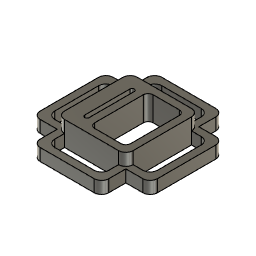
tv-foot-crt (Autodesk Fusion 360 design; units mm, degrees)
Autodesk Fusion 360 part; units mm, degrees
sketch "Sketch1" plane through (0, 0, 0) normal (0, 0, 1) x (1, 0, 0)
  line L0 (0, 0) -> (70.5, 0)
  line L1 (70.5, 0) -> (70.5, 75)
  line L2 (70.5, 75) -> (0, 75)
  line L3 (0, 75) -> (0, 0)
  line L4 (70.5, 0) -> (415.5625, 0) construction
  line L5 (16.25, 75) -> (16.25, 0) construction
  line L6 (14, 60.75) -> (14, 14.25)
  arc A0 (14, 14.25) -> (18.5, 14.25) centre (16.25, 14.25) ccw
  line L7 (18.5, 14.25) -> (18.5, 60.75)
  arc A1 (18.5, 60.75) -> (14, 60.75) centre (16.25, 60.75) ccw
  line L8 (16.25, 63) -> (16.25, 12) construction
  line L9 (12, 60.75) -> (12, 14.25)
  arc A2 (12, 14.25) -> (20.5, 14.25) centre (16.25, 14.25) ccw
  line L10 (20.5, 14.25) -> (20.5, 60.75)
  arc A3 (20.5, 60.75) -> (12, 60.75) centre (16.25, 60.75) ccw
  line L11 (8, 0) -> (8, 75)
  dimension "d3" = 75
  dimension "d10" = 4.5
  dimension "d13" = 2
  dimension "d14" = 10
  dimension "d15" = 10
  dimension "d21" = 8
  dimension "d23" = 4
  dimension "d39" = 50
  constraint coincident L0.start L3.end
  constraint horizontal L0
  constraint vertical L1
  constraint horizontal L2
  constraint vertical L3
  constraint perpendicular L1 L4
  constraint coincident L2 L5.start
  constraint coincident L0 L5.end
  constraint perpendicular L0 L5
  constraint tangent L6 A0
  constraint tangent A0 L7
  constraint parallel L6 L7
  constraint tangent L7 A1
  constraint tangent L6 A1
  constraint midpoint A1 L8.start
  constraint midpoint A0 L8.end
  constraint coincident L5 L8.end
  constraint parallel L5 L8
  constraint coincident L0 L11.start
  constraint coincident L2 L11.end
  constraint perpendicular L2 L11
  measures "d3" distance of L0.end L1.end
  measures "d10" distance of L6 L7
  measures "d14" distance of L2 A3
  measures "d15" distance of L0 A2
  measures "d21" distance of L3 L11
  measures "d23" distance of L9 L11
  measures "d39" distance of L1 L10
extrude "Extrude1" add sketch "Sketch1" along normal blind 25 contours L0 L2 L3 L11 | L0 L1 L2 L11 | L9 A2 L10 A3
extrude "Extrude2" cut sketch "Sketch1" against normal up to surface (20 mm away) from surface at 20 contours L9 A2 L10 A3
sketch "Sketch3" plane through (0, 75, 0) normal (0, 1, 0) x (-1, 0, 0)
  line L0 (-70.5, 0) -> (0, 0)
  line L1 (0, 0) -> (0, 25)
  line L2 (0, 25) -> (-70.5, 25)
  line L3 (-70.5, 25) -> (-70.5, 0)
  line L4 (-70.5, 12.5) -> (0, 12.5)
  constraint midpoint L3 L4.start
  constraint midpoint L1 L4.end
extrude "Extrude5" add sketch "Sketch3" along normal blind 25 contours L0 L1 L3 L4
extrude "Extrude6" add 1 faces at (47, 100, 8.3333) along direction (0, -1, 0) blind 25 from surface at 100
sketch "Sketch4" plane through (0, 0, 25) normal (0, 0, 1) x (-1, 0, 0)
  arc A0 (-18.5, -60.75) -> (-14, -60.75) centre (-16.25, -60.75) ccw
  line L0 (-18.5, -60.75) -> (-18.5, -14.25)
  arc A1 (-14, -14.25) -> (-18.5, -14.25) centre (-16.25, -14.25) ccw
  line L1 (-14, -14.25) -> (-14, -60.75)
  line L2 (0, -75) -> (0, 0)
  line L3 (0, 0) -> (-70.5, 0)
  line L4 (-70.5, 0) -> (-70.5, -75)
  line L5 (-70.5, -75) -> (0, -75)
  line L6 (-70.5, -75) -> (-70.5, -100)
  line L7 (-70.5, -75) -> (0, -75)
  line L8 (0, -75) -> (0, -100)
  line L9 (0, -100) -> (-70.5, -100)
  line L10 (-70.5, 0) -> (-70.5, -75)
  line L11 (-18.5, -60.75) -> (-18.5, -14.25)
  line L12 (-70.5, -37.5) -> (-18.5, -37.5) construction
  line L13 (-63, -75) -> (-63, -92.5)
  line L14 (-7.5, -92.5) -> (-63, -92.5)
  line L15 (-7.5, -75) -> (-7.5, -92.5)
  line L16 (-63, 0) -> (-63, 17.5)
  line L17 (-7.5, 17.5) -> (-63, 17.5)
  line L18 (-7.5, 0) -> (-7.5, 17.5)
  line L19 (-26, -37.5) -> (-26, -67.5)
  line L20 (-26, -67.5) -> (-63, -67.5)
  line L21 (-63, -67.5) -> (-63, -37.5)
  line L22 (-26, -37.5) -> (-26, -7.5)
  line L23 (-26, -7.5) -> (-63, -7.5)
  line L24 (-63, -7.5) -> (-63, -37.5)
  dimension "d58" = -7.5
  dimension "d67" = 7.5
  dimension "d68" = 7.5
  dimension "d69" = 7.5
  constraint midpoint L10 L12.start
  constraint midpoint L11 L12.end
  constraint symmetric L12 L13.start L16.start
  constraint symmetric L12 L13.end L16.end
  constraint symmetric L12 L14.start L17.start
  constraint symmetric L12 L15.start L18.start
  constraint coincident L12 L19.start
  constraint perpendicular L12 L19
  constraint perpendicular L19 L20
  constraint coincident L12 L21.end
  constraint perpendicular L12 L21
  constraint symmetric L12 L19.start L22.start
  constraint symmetric L12 L19.end L22.end
  constraint symmetric L12 L20.end L23.end
  constraint symmetric L12 L21.end L24.end
  measures "d67" distance of L0 L19
  measures "d68" distance of L4 L21
  measures "d69" distance of L7 L20
extrude "Extrude7" cut sketch "Sketch4" against normal up to surface (12.5 mm away) from surface at -12.5 contours L5 L7 L13 L14 L15 | L3 L16 L17 L18
fillet "Fillet8" radius 7.5 4 edges at (70.5, 100, 6.25) (0, 100, 6.25) (70.5, -25, 6.25) (0, -25, 6.25)
fillet "Fillet8" radius 7.5 4 edges at (7.5, -17.5, 6.25) (7.5, 92.5, 6.25) (63, 92.5, 6.25) (63, -17.5, 6.25)
extrude "Extrude8" cut sketch "Sketch4" against normal up to surface (25 mm away) contours L19 L20 L21 L22 L23 L24
fillet "Fillet9" radius 5 4 edges at (63, 7.5, 12.5) (63, 67.5, 12.5) (26, 67.5, 12.5) (26, 7.5, 12.5)
sketch "Sketch5" plane through (70.5, 0, 0) normal (1, 0, 0) x (0, 1, 0)
  line L0 (92.5, 12.5) -> (75, 12.5)
  line L1 (75, 25) -> (0, 25)
  line L2 (0, 12.5) -> (-17.5, 12.5)
  line L3 (-17.5, 12.5) -> (-17.5, 0)
  line L4 (-17.5, 0) -> (92.5, 0)
  line L5 (92.5, 0) -> (92.5, 12.5)
  line L6 (0, 12.5) -> (-17.5, 12.5)
  line L7 (75, 12.5) -> (92.5, 12.5)
  line L8 (0, 12.5) -> (75, 12.5)
  line L9 (37.5, 12.5) -> (37.5, 0) construction
  line L10 (0, 12.5) -> (0, 0)
  line L11 (75, 12.5) -> (75, 0)
  line L12 (75, 12.5) -> (75, 25)
  line L13 (0, 25) -> (0, 12.5)
  constraint coincident L2.start L6.start
  constraint coincident L0.end L7.start
  constraint midpoint L8 L9.start
  constraint midpoint L4 L9.end
  constraint coincident L4 L10.end
  constraint perpendicular L4 L10
  constraint coincident L4 L11.end
  constraint perpendicular L4 L11
extrude "Extrude9" add sketch "Sketch5" along normal blind 25 contours L4 L8 L10 L11
extrude "Extrude10" add 1 faces at (95.5, 25, 8.3333) along direction (-1, 0, 0) blind 25 from surface at 95.5
sketch "Sketch7" plane through (0, 0, 25) normal (0, 0, 1) x (-1, 0, 0)
  line L0 (-31, -67.5) -> (-58, -67.5)
  arc A0 (-63, -62.5) -> (-58, -67.5) centre (-58, -62.5) ccw
  line L1 (-63, -62.5) -> (-63, -12.5)
  arc A1 (-58, -7.5) -> (-63, -12.5) centre (-58, -12.5) ccw
  line L2 (-58, -7.5) -> (-31, -7.5)
  arc A2 (-26, -12.5) -> (-31, -7.5) centre (-31, -12.5) ccw
  line L3 (-26, -12.5) -> (-26, -62.5)
  arc A3 (-31, -67.5) -> (-26, -62.5) centre (-31, -62.5) ccw
  arc A4 (-18.5, -60.75) -> (-14, -60.75) centre (-16.25, -60.75) ccw
  line L4 (-18.5, -60.75) -> (-18.5, -14.25)
  arc A5 (-14, -14.25) -> (-18.5, -14.25) centre (-16.25, -14.25) ccw
  line L5 (-14, -14.25) -> (-14, -60.75)
  line L6 (0, -75) -> (0, 0)
  line L7 (0, 0) -> (-70.5, 0)
  line L8 (-70.5, 0) -> (-70.5, -75)
  line L9 (-70.5, -75) -> (0, -75)
  line L10 (0, -75) -> (0, 0)
  line L11 (-70.5, 0) -> (-70.5, -75)
  line L12 (-35.25, 0) -> (-35.25, -75) construction
  line L13 (-70.5, -67.5) -> (-88, -67.5)
  line L14 (-88, -67.5) -> (-88, -7.5)
  line L15 (-88, -7.5) -> (-70.5, -7.5)
  line L16 (-70.5, -75) -> (-95.5, -75)
  line L17 (-95.5, -75) -> (-95.5, 0)
  line L18 (-70.5, 0) -> (-95.5, 0)
  line L19 (0, -67.5) -> (17.5, -67.5)
  line L20 (17.5, -67.5) -> (17.5, -7.5)
  line L21 (17.5, -7.5) -> (0, -7.5)
  dimension "d108" = 7.5
  dimension "d109" = 7.5
  dimension "d110" = 7.5
  constraint midpoint L7 L12.start
  constraint midpoint L9 L12.end
  constraint coincident L11 L13.start
  constraint perpendicular L11 L13
  constraint perpendicular L13 L14
  constraint coincident L11 L15.end
  constraint perpendicular L11 L15
  constraint symmetric L12 L13.start L19.start
  constraint symmetric L12 L13.end L19.end
  constraint symmetric L12 L14.end L20.end
  constraint symmetric L12 L15.end L21.end
  measures "d108" distance of L13 L16
  measures "d109" distance of L14 L17
  measures "d110" distance of L15 L18
extrude "Extrude12" cut sketch "Sketch7" against normal up to surface (25 mm away) contours L6 L10 L19 L20 L21 | L8 L11 L13 L14 L15
fillet "Fillet16" radius 7.5 4 edges at (88, 67.5, 6.25) (88, 7.5, 6.25) (-17.5, 7.5, 6.25) (-17.5, 67.5, 6.25)
fillet "Fillet17" radius 7.5 4 edges at (95.5, 0, 6.25) (95.5, 75, 6.25) (-25, 75, 6.25) (-25, 0, 6.25)
fillet "Fillet18" radius 7.5 4 edges at (70.5, 0, 18.75) (0, 0, 18.75) (70.5, 75, 18.75) (0, 75, 18.75)
named bodies: "tv-foot-crt"
